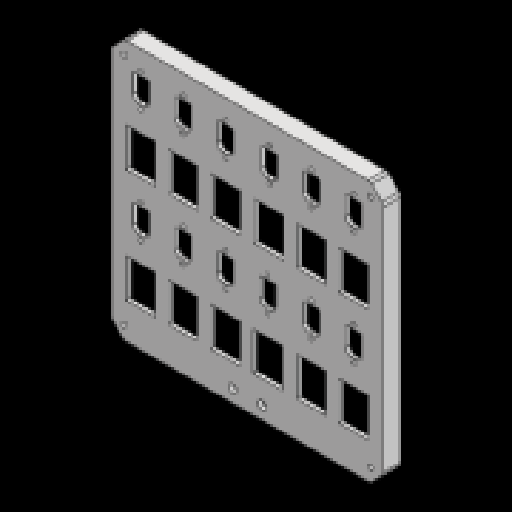
# Autodesk Inventor part: PowerHub
Saved by Autodesk Inventor 2025.2 (Build 292293000, 293)
## iProperties
Created: 2026-06-06
Part Number: PowerHub
Material: Generic
Document SubType Name: Modeling
Designer: valer
Density: 1 g/cm^3
Appearance: Default
Author: valer
Autodesk Inventor part; units mm, degrees
(part 1 of 2)
ref_plane "YZ Plane" through (0, 0, 0) normal (1, 0, 0) x (0, 1, 0)
ref_plane "XZ Plane" through (0, 0, 0) normal (0, 1, 0) x (-1, 0, 0)
ref_plane "XY Plane" through (0, 0, 0) normal (0, 0, 1) x (1, 0, 0)
sketch "Panel" plane through (0, 0, 0) normal (0, 0, 1) x (1, 0, 0)
  line L0 (-102.5, -98.125) -> (102.5, -98.125)
  line L1 (102.5, -98.125) -> (102.5, 98.125)
  line L2 (102.5, 98.125) -> (-102.5, 98.125)
  line L3 (-102.5, 98.125) -> (-102.5, -98.125)
  line L4 (-102.5, -98.125) -> (102.5, 98.125) construction
  line L5 (102.5, -98.125) -> (-102.5, 98.125) construction
  line L6 (-143.5, 0) -> (143.5, 0) construction
  line L7 (0, -137.375) -> (0, 137.375) construction
  line L8 (-88, 88.125) -> (-72, 88.125)
  line L9 (-72, 88.125) -> (-72, 54.125)
  line L10 (-72, 54.125) -> (-88, 54.125)
  line L11 (-88, 54.125) -> (-88, 88.125)
  line L12 (-80, 88.125) -> (-80, 12.875) construction
  line L13 (-92.5, 44.375) -> (-67.5, 44.375)
  line L14 (-67.5, 44.375) -> (-67.5, 12.875)
  line L15 (-67.5, 12.875) -> (-92.5, 12.875)
  line L16 (-92.5, 12.875) -> (-92.5, 44.375)
  line L17 (-56, 88.125) -> (-40, 88.125)
  line L18 (-56, 54.125) -> (-56, 88.125)
  line L19 (-40, 88.125) -> (-40, 54.125)
  line L20 (-40, 54.125) -> (-56, 54.125)
  line L21 (-60.5, 44.375) -> (-35.5, 44.375)
  line L22 (-60.5, 12.875) -> (-60.5, 44.375)
  line L23 (-35.5, 44.375) -> (-35.5, 12.875)
  line L24 (-35.5, 12.875) -> (-60.5, 12.875)
  line L25 (-24, 88.125) -> (-8, 88.125)
  line L26 (-24, 54.125) -> (-24, 88.125)
  line L27 (-8, 88.125) -> (-8, 54.125)
  line L28 (-8, 54.125) -> (-24, 54.125)
  line L29 (-28.5, 44.375) -> (-3.5, 44.375)
  line L30 (-28.5, 12.875) -> (-28.5, 44.375)
  line L31 (-3.5, 44.375) -> (-3.5, 12.875)
  line L32 (-3.5, 12.875) -> (-28.5, 12.875)
  line L33 (8, 88.125) -> (24, 88.125)
  line L34 (8, 54.125) -> (8, 88.125)
  line L35 (24, 88.125) -> (24, 54.125)
  line L36 (24, 54.125) -> (8, 54.125)
  line L37 (3.5, 44.375) -> (28.5, 44.375)
  line L38 (3.5, 12.875) -> (3.5, 44.375)
  line L39 (28.5, 44.375) -> (28.5, 12.875)
  line L40 (28.5, 12.875) -> (3.5, 12.875)
  line L41 (40, 88.125) -> (56, 88.125)
  line L42 (40, 54.125) -> (40, 88.125)
  line L43 (56, 88.125) -> (56, 54.125)
  line L44 (56, 54.125) -> (40, 54.125)
  line L45 (35.5, 44.375) -> (60.5, 44.375)
  line L46 (35.5, 12.875) -> (35.5, 44.375)
  line L47 (60.5, 44.375) -> (60.5, 12.875)
  line L48 (60.5, 12.875) -> (35.5, 12.875)
  line L49 (72, 88.125) -> (88, 88.125)
  line L50 (72, 54.125) -> (72, 88.125)
  line L51 (88, 88.125) -> (88, 54.125)
  line L52 (88, 54.125) -> (72, 54.125)
  line L53 (67.5, 44.375) -> (92.5, 44.375)
  line L54 (67.5, 12.875) -> (67.5, 44.375)
  line L55 (92.5, 44.375) -> (92.5, 12.875)
  line L56 (92.5, 12.875) -> (67.5, 12.875)
  line L57 (-88, 3.125) -> (-72, 3.125)
  line L58 (-88, -30.875) -> (-88, 3.125)
  line L59 (-72, 3.125) -> (-72, -30.875)
  line L60 (-72, -30.875) -> (-88, -30.875)
  line L61 (-92.5, -40.625) -> (-67.5, -40.625)
  line L62 (-92.5, -72.125) -> (-92.5, -40.625)
  line L63 (-67.5, -40.625) -> (-67.5, -72.125)
  line L64 (-67.5, -72.125) -> (-92.5, -72.125)
  line L65 (-56, 3.125) -> (-40, 3.125)
  line L66 (-56, -30.875) -> (-56, 3.125)
  line L67 (-40, 3.125) -> (-40, -30.875)
  line L68 (-40, -30.875) -> (-56, -30.875)
  line L69 (-60.5, -40.625) -> (-35.5, -40.625)
  line L70 (-60.5, -72.125) -> (-60.5, -40.625)
  line L71 (-35.5, -40.625) -> (-35.5, -72.125)
  line L72 (-35.5, -72.125) -> (-60.5, -72.125)
  line L73 (-24, 3.125) -> (-8, 3.125)
  line L74 (-24, -30.875) -> (-24, 3.125)
  line L75 (-8, 3.125) -> (-8, -30.875)
  line L76 (-8, -30.875) -> (-24, -30.875)
  line L77 (-28.5, -40.625) -> (-3.5, -40.625)
  line L78 (-28.5, -72.125) -> (-28.5, -40.625)
  line L79 (-3.5, -40.625) -> (-3.5, -72.125)
  line L80 (-3.5, -72.125) -> (-28.5, -72.125)
  line L81 (8, 3.125) -> (24, 3.125)
  line L82 (8, -30.875) -> (8, 3.125)
  line L83 (24, 3.125) -> (24, -30.875)
  line L84 (24, -30.875) -> (8, -30.875)
  line L85 (3.5, -40.625) -> (28.5, -40.625)
  line L86 (3.5, -72.125) -> (3.5, -40.625)
  line L87 (28.5, -40.625) -> (28.5, -72.125)
  line L88 (28.5, -72.125) -> (3.5, -72.125)
  line L89 (40, 3.125) -> (56, 3.125)
  line L90 (40, -30.875) -> (40, 3.125)
  line L91 (56, 3.125) -> (56, -30.875)
  line L92 (56, -30.875) -> (40, -30.875)
  line L93 (35.5, -40.625) -> (60.5, -40.625)
  line L94 (35.5, -72.125) -> (35.5, -40.625)
  line L95 (60.5, -40.625) -> (60.5, -72.125)
  line L96 (60.5, -72.125) -> (35.5, -72.125)
  line L97 (72, 3.125) -> (88, 3.125)
  line L98 (72, -30.875) -> (72, 3.125)
  line L99 (88, 3.125) -> (88, -30.875)
  line L100 (88, -30.875) -> (72, -30.875)
  line L101 (67.5, -40.625) -> (92.5, -40.625)
  line L102 (67.5, -72.125) -> (67.5, -40.625)
  line L103 (92.5, -40.625) -> (92.5, -72.125)
  line L104 (92.5, -72.125) -> (67.5, -72.125)
  line L105 (-11, -88.625) -> (11, -88.625) construction
  circle A0 centre (-11, -88.625) radius 3.2
  circle A1 centre (11, -88.625) radius 3.2
  line L106 (-20.5, -98.125) -> (-1.5, -98.125)
  line L107 (-1.5, -98.125) -> (-1.5, -79.125)
  line L108 (-1.5, -79.125) -> (-20.5, -79.125)
  line L109 (-20.5, -79.125) -> (-20.5, -98.125)
  line L110 (-20.5, -98.125) -> (-1.5, -79.125) construction
  line L111 (-1.5, -98.125) -> (-20.5, -79.125) construction
  line L112 (1.5, -98.125) -> (20.5, -98.125)
  line L113 (20.5, -98.125) -> (20.5, -79.125)
  line L114 (20.5, -79.125) -> (1.5, -79.125)
  line L115 (1.5, -79.125) -> (1.5, -98.125)
  line L116 (1.5, -98.125) -> (20.5, -79.125) construction
  line L117 (20.5, -98.125) -> (1.5, -79.125) construction
  line L118 (-22.5, -77.125) -> (22.5, -77.125)
  line L119 (22.5, -77.125) -> (22.5, -98.125)
  line L120 (22.5, -98.125) -> (-22.5, -98.125)
  line L121 (-22.5, -98.125) -> (-22.5, -77.125)
  point P0 (0, 0)
  point P1 (-48, 88.125)
  point P2 (-48, 12.875)
  point P3 (-16, 88.125)
  point P4 (-16, 12.875)
  point P5 (16, 88.125)
  point P6 (16, 12.875)
  point P7 (48, 88.125)
  point P8 (48, 12.875)
  point P9 (80, 88.125)
  point P10 (80, 12.875)
  point P11 (-80, 3.125)
  point P12 (-80, -72.125)
  point P13 (-48, 3.125)
  point P14 (-48, -72.125)
  point P15 (-16, 3.125)
  point P16 (-16, -72.125)
  point P17 (16, 3.125)
  point P18 (16, -72.125)
  point P19 (48, 3.125)
  point P20 (48, -72.125)
  point P21 (80, 3.125)
  point P22 (80, -72.125)
  point P23 (0, -88.625)
  dimension "d0" = 16
  dimension "d1" = 34
  dimension "d2" = 25
  dimension "d3" = 31.5
  dimension "d4" = 9.75
  dimension "d5" = 10
  dimension "d6" = 10
  dimension "d9" = 32
  dimension "d12" = 85
  dimension "d15" = 10
  dimension "d16" = 9.75
  dimension "d17" = 22
  dimension "d18" = 6.4
  dimension "d19" = 19
  dimension "d24" = 2
  dimension "d25" = 2
  dimension "d26" = 2
  dimension "d27" = 5
  dimension "d37" = 16
  dimension "d38" = 14.5
  constraints: 240 end point, 12 parallel, 9 midpoint, 8 horizontal, 7 perpendicular, 4 collinear, 3 equal length, 2 centre point, 2 coincident, 1 equal radius, 1 point on line, 1 vertical, 196 other
  measures "d0" distance of L8.start L8.end
  measures "d1" distance of L8.end L9.end
  measures "d2" distance of L14.end L15.end
  measures "d3" distance of L13.end L14.end
  measures "d4" distance between parallel lines of L13 L10
  measures "d5" distance between parallel lines of L3 L16
  measures "d6" distance between parallel lines of L2 L8
  measures "d9" distance of L8.start L17.start
  measures "d12" distance of L8.start L57.start
  measures "d15" distance between parallel lines of L1 L55
  measures "d16" distance between parallel lines of L57 L15
  measures "d17" distance of L105.start L105.end
  measures "d18" diameter of A0
  measures "d19" distance of L107.end L108.end
  measures "d24" distance between parallel lines of L118 L114
  measures "d25" distance between parallel lines of L119 L113
  measures "d26" distance between parallel lines of L109 L121
  measures "d27" distance between parallel lines of L118 L80
  measures "d37" distance between parallel lines of L18 L9
  measures "d38" distance between parallel lines of L3 L11
extrude "PanelFeature" add sketch "Panel" along normal blind 3 contours L3 L2 L1 L0 L119 L118 L121 | L121 L118 L119 L0 L113 L114 L115 L107 L108 L109 | L109 L108 L107 L0 | L115 L114 L113 L0 | L8 L9 L10 L11 | L13 L14 L15 L16 | L17 L19 L20 L18 | L21 L23 L24 L22 | L25 L27 L28 L26 | L29 L31 L32 L30 | L33 L35 L36 L34 | L37 L39 L40 L38 | L41 L43 L44 L42 | L45 L47 L48 L46 | L49 L51 L52 L50 | L53 L55 L56 L54 | L57 L59 L60 L58 | L61 L63 L64 L62 | L65 L67 L68 L66 | L69 L71 L72 L70 | L73 L75 L76 L74 | L77 L79 L80 L78 | L81 L83 L84 L82 | L85 L87 L88 L86 | L89 L91 L92 L90 | L93 L95 L96 L94 | L97 L99 L100 L98 | L101 L103 L104 L102
chamfer "OutsideChamfersFeature" distance 10 angle 45 4 edges at (-102.5, 98.125, 1.5) (-102.5, -98.125, 1.5) (102.5, -98.125, 1.5) (102.5, 98.125, 1.5)
fillet "FilletsFeature" radius 4 8 edges at (-92.5, -98.125, 1.5) (-102.5, -88.125, 1.5) (92.5, -98.125, 1.5) (102.5, -88.125, 1.5) (92.5, 98.125, 1.5) (102.5, 88.125, 1.5) (-102.5, 88.125, 1.5) (-92.5, 98.125, 1.5)
sketch "MountHoles" plane through (0, 0, 3) normal (0, 0, 1) x (1, 0, 0)
  arc A0 (-90.8431, 98.125) -> (-93.6716, 96.9534) centre (-90.8431, 94.125) ccw projected
  line L0 (-101.3284, 89.2966) -> (-93.6716, 96.9534) projected
  arc A1 (-101.3284, 89.2966) -> (-102.5, 86.4681) centre (-98.5, 86.4681) ccw projected
  line L1 (-102.5, 86.4681) -> (-102.5, -86.4681) projected
  arc A2 (-102.5, -86.4681) -> (-101.3284, -89.2966) centre (-98.5, -86.4681) ccw projected
  line L2 (-93.6716, -96.9534) -> (-101.3284, -89.2966) projected
  arc A3 (-93.6716, -96.9534) -> (-90.8431, -98.125) centre (-90.8431, -94.125) ccw projected
  line L3 (-90.8431, -98.125) -> (90.8431, -98.125) projected
  arc A4 (90.8431, -98.125) -> (93.6716, -96.9534) centre (90.8431, -94.125) ccw projected
  line L4 (101.3284, -89.2966) -> (93.6716, -96.9534) projected
  arc A5 (101.3284, -89.2966) -> (102.5, -86.4681) centre (98.5, -86.4681) ccw projected
  line L5 (102.5, -86.4681) -> (102.5, 86.4681) projected
  arc A6 (102.5, 86.4681) -> (101.3284, 89.2966) centre (98.5, 86.4681) ccw projected
  line L6 (93.6716, 96.9534) -> (101.3284, 89.2966) projected
  arc A7 (93.6716, 96.9534) -> (90.8431, 98.125) centre (90.8431, 94.125) ccw projected
  line L7 (90.8431, 98.125) -> (-90.8431, 98.125) projected
  circle A8 centre (-92.5, 88.125) radius 2
  line L8 (-143.8938, 0) -> (143.8938, 0) projected
  line L9 (0, -137.7688) -> (0, 137.7688) projected
  circle A9 centre (92.5, 88.125) radius 2
  circle A10 centre (-92.5, -88.125) radius 2
  circle A11 centre (92.5, -88.125) radius 2
  point P0 (0, 0)
  dimension "d32" = 4
  dimension "d33" = 10
  dimension "d34" = 10
  constraints: 4 centre point, 3 symmetric about line, 3 other
  measures "d32" diameter of A8
  measures "d33" distance from line of L7 A8.centre
  measures "d34" distance from line of L1 A8.centre
extrude "MountHolesFeature" cut sketch "MountHoles" against normal through all contours A8 | A9 | A10 | A11
sketch "ThroughHoles" plane through (0, 0, 0) normal (0, 0, -1) x (-1, 0, 0)
  circle A0 centre (-80.1, 67.625) radius 2.5 projected
  circle A1 centre (-80.1, 74.625) radius 2.5 projected
  arc A2 (-86, 65.675) -> (-82.2, 61.875) centre (-82.2, 65.675) ccw projected
  line L0 (-82.2, 61.875) -> (-78, 61.875) projected
  arc A3 (-78, 61.875) -> (-74.2, 65.675) centre (-78, 65.675) ccw projected
  line L1 (-74.2, 65.675) -> (-74.2, 79.375) projected
  arc A4 (-74.2, 79.375) -> (-75.2, 80.375) centre (-75.2, 79.375) ccw projected
  line L2 (-75.2, 80.375) -> (-85, 80.375) projected
  arc A5 (-85, 80.375) -> (-86, 79.375) centre (-85, 79.375) ccw projected
  line L3 (-86, 79.375) -> (-86, 65.675) projected
  circle A6 centre (-48.3, 67.625) radius 2.5 projected
  circle A7 centre (-48.3, 74.625) radius 2.5 projected
  arc A8 (-54.2, 65.675) -> (-50.4, 61.875) centre (-50.4, 65.675) ccw projected
  line L4 (-50.4, 61.875) -> (-46.2, 61.875) projected
  arc A9 (-46.2, 61.875) -> (-42.4, 65.675) centre (-46.2, 65.675) ccw projected
  line L5 (-42.4, 65.675) -> (-42.4, 79.375) projected
  arc A10 (-42.4, 79.375) -> (-43.4, 80.375) centre (-43.4, 79.375) ccw projected
  line L6 (-43.4, 80.375) -> (-53.2, 80.375) projected
  arc A11 (-53.2, 80.375) -> (-54.2, 79.375) centre (-53.2, 79.375) ccw projected
  line L7 (-54.2, 79.375) -> (-54.2, 65.675) projected
  circle A12 centre (-16.5, 67.625) radius 2.5 projected
  circle A13 centre (-16.5, 74.625) radius 2.5 projected
  arc A14 (-22.4, 65.675) -> (-18.6, 61.875) centre (-18.6, 65.675) ccw projected
  line L8 (-18.6, 61.875) -> (-14.4, 61.875) projected
  arc A15 (-14.4, 61.875) -> (-10.6, 65.675) centre (-14.4, 65.675) ccw projected
  line L9 (-10.6, 65.675) -> (-10.6, 79.375) projected
  arc A16 (-10.6, 79.375) -> (-11.6, 80.375) centre (-11.6, 79.375) ccw projected
  line L10 (-11.6, 80.375) -> (-21.4, 80.375) projected
  arc A17 (-21.4, 80.375) -> (-22.4, 79.375) centre (-21.4, 79.375) ccw projected
  line L11 (-22.4, 79.375) -> (-22.4, 65.675) projected
  circle A18 centre (16.5, 67.625) radius 2.5 projected
  circle A19 centre (16.5, 74.625) radius 2.5 projected
  arc A20 (10.6, 65.675) -> (14.4, 61.875) centre (14.4, 65.675) ccw projected
  line L12 (14.4, 61.875) -> (18.6, 61.875) projected
  arc A21 (18.6, 61.875) -> (22.4, 65.675) centre (18.6, 65.675) ccw projected
  line L13 (22.4, 65.675) -> (22.4, 79.375) projected
  arc A22 (22.4, 79.375) -> (21.4, 80.375) centre (21.4, 79.375) ccw projected
  line L14 (21.4, 80.375) -> (11.6, 80.375) projected
  arc A23 (11.6, 80.375) -> (10.6, 79.375) centre (11.6, 79.375) ccw projected
  line L15 (10.6, 79.375) -> (10.6, 65.675) projected
  circle A24 centre (48.3, 67.625) radius 2.5 projected
  circle A25 centre (48.3, 74.625) radius 2.5 projected
  arc A26 (42.4, 65.675) -> (46.2, 61.875) centre (46.2, 65.675) ccw projected
  line L16 (46.2, 61.875) -> (50.4, 61.875) projected
  arc A27 (50.4, 61.875) -> (54.2, 65.675) centre (50.4, 65.675) ccw projected
  line L17 (54.2, 65.675) -> (54.2, 79.375) projected
  arc A28 (54.2, 79.375) -> (53.2, 80.375) centre (53.2, 79.375) ccw projected
  line L18 (53.2, 80.375) -> (43.4, 80.375) projected
  arc A29 (43.4, 80.375) -> (42.4, 79.375) centre (43.4, 79.375) ccw projected
  line L19 (42.4, 79.375) -> (42.4, 65.675) projected
  circle A30 centre (80.1, 67.625) radius 2.5 projected
  circle A31 centre (80.1, 74.625) radius 2.5 projected
  arc A32 (74.2, 65.675) -> (78, 61.875) centre (78, 65.675) ccw projected
  line L20 (78, 61.875) -> (82.2, 61.875) projected
  arc A33 (82.2, 61.875) -> (86, 65.675) centre (82.2, 65.675) ccw projected
  line L21 (86, 65.675) -> (86, 79.375) projected
  arc A34 (86, 79.375) -> (85, 80.375) centre (85, 79.375) ccw projected
  line L22 (85, 80.375) -> (75.2, 80.375) projected
  arc A35 (75.2, 80.375) -> (74.2, 79.375) centre (75.2, 79.375) ccw projected
  line L23 (74.2, 79.375) -> (74.2, 65.675) projected
  line L24 (73.4544, 40.127) -> (86.7456, 40.127) projected
  line L25 (86.7456, 40.127) -> (86.7456, 17.127) projected
  line L26 (86.7456, 17.127) -> (73.4544, 17.127) projected
  line L27 (73.4544, 17.127) -> (73.4544, 40.127) projected
  line L28 (90.895, 42.851) -> (69.305, 42.851) projected
  line L29 (69.305, 42.851) -> (69.305, 14.403) projected
  line L30 (69.305, 14.403) -> (90.895, 14.403) projected
  line L31 (90.895, 14.403) -> (90.895, 42.851) projected
  line L32 (41.6544, 40.127) -> (54.9456, 40.127) projected
  line L33 (54.9456, 40.127) -> (54.9456, 17.127) projected
  line L34 (54.9456, 17.127) -> (41.6544, 17.127) projected
  line L35 (41.6544, 17.127) -> (41.6544, 40.127) projected
  line L36 (59.095, 42.851) -> (37.505, 42.851) projected
  line L37 (37.505, 42.851) -> (37.505, 14.403) projected
  line L38 (37.505, 14.403) -> (59.095, 14.403) projected
  line L39 (59.095, 14.403) -> (59.095, 42.851) projected
  line L40 (9.8544, 40.127) -> (23.1456, 40.127) projected
  line L41 (23.1456, 40.127) -> (23.1456, 17.127) projected
  line L42 (23.1456, 17.127) -> (9.8544, 17.127) projected
  line L43 (9.8544, 17.127) -> (9.8544, 40.127) projected
  line L44 (27.295, 42.851) -> (5.705, 42.851) projected
  line L45 (5.705, 42.851) -> (5.705, 14.403) projected
  line L46 (5.705, 14.403) -> (27.295, 14.403) projected
  line L47 (27.295, 14.403) -> (27.295, 42.851) projected
  line L48 (-23.1456, 40.127) -> (-9.8544, 40.127) projected
  line L49 (-9.8544, 40.127) -> (-9.8544, 17.127) projected
  line L50 (-9.8544, 17.127) -> (-23.1456, 17.127) projected
  line L51 (-23.1456, 17.127) -> (-23.1456, 40.127) projected
  line L52 (-5.705, 42.851) -> (-27.295, 42.851) projected
  line L53 (-27.295, 42.851) -> (-27.295, 14.403) projected
  line L54 (-27.295, 14.403) -> (-5.705, 14.403) projected
  line L55 (-5.705, 14.403) -> (-5.705, 42.851) projected
  line L56 (-54.9456, 40.127) -> (-41.6544, 40.127) projected
  line L57 (-41.6544, 40.127) -> (-41.6544, 17.127) projected
  line L58 (-41.6544, 17.127) -> (-54.9456, 17.127) projected
  line L59 (-54.9456, 17.127) -> (-54.9456, 40.127) projected
  line L60 (-37.505, 42.851) -> (-59.095, 42.851) projected
  line L61 (-59.095, 42.851) -> (-59.095, 14.403) projected
  line L62 (-59.095, 14.403) -> (-37.505, 14.403) projected
  line L63 (-37.505, 14.403) -> (-37.505, 42.851) projected
  line L64 (-86.7456, 40.127) -> (-73.4544, 40.127) projected
  line L65 (-73.4544, 40.127) -> (-73.4544, 17.127) projected
  line L66 (-73.4544, 17.127) -> (-86.7456, 17.127) projected
  line L67 (-86.7456, 17.127) -> (-86.7456, 40.127) projected
  line L68 (-69.305, 42.851) -> (-90.895, 42.851) projected
  line L69 (-90.895, 42.851) -> (-90.895, 14.403) projected
  line L70 (-90.895, 14.403) -> (-69.305, 14.403) projected
  line L71 (-69.305, 14.403) -> (-69.305, 42.851) projected
  circle A36 centre (-80.1, -17.621) radius 2.5 projected
  circle A37 centre (-80.1, -10.621) radius 2.5 projected
  arc A38 (-86, -19.571) -> (-82.2, -23.371) centre (-82.2, -19.571) ccw projected
  line L72 (-82.2, -23.371) -> (-78, -23.371) projected
  arc A39 (-78, -23.371) -> (-74.2, -19.571) centre (-78, -19.571) ccw projected
  line L73 (-74.2, -19.571) -> (-74.2, -5.871) projected
  arc A40 (-74.2, -5.871) -> (-75.2, -4.871) centre (-75.2, -5.871) ccw projected
  line L74 (-75.2, -4.871) -> (-85, -4.871) projected
  arc A41 (-85, -4.871) -> (-86, -5.871) centre (-85, -5.871) ccw projected
  line L75 (-86, -5.871) -> (-86, -19.571) projected
  circle A42 centre (-48.3, -17.621) radius 2.5 projected
  circle A43 centre (-48.3, -10.621) radius 2.5 projected
  arc A44 (-54.2, -19.571) -> (-50.4, -23.371) centre (-50.4, -19.571) ccw projected
  line L76 (-50.4, -23.371) -> (-46.2, -23.371) projected
  arc A45 (-46.2, -23.371) -> (-42.4, -19.571) centre (-46.2, -19.571) ccw projected
  line L77 (-42.4, -19.571) -> (-42.4, -5.871) projected
  arc A46 (-42.4, -5.871) -> (-43.4, -4.871) centre (-43.4, -5.871) ccw projected
  line L78 (-43.4, -4.871) -> (-53.2, -4.871) projected
  arc A47 (-53.2, -4.871) -> (-54.2, -5.871) centre (-53.2, -5.871) ccw projected
  line L79 (-54.2, -5.871) -> (-54.2, -19.571) projected
  circle A48 centre (-15.3, -17.621) radius 2.5 projected
  circle A49 centre (-15.3, -10.621) radius 2.5 projected
  arc A50 (-21.2, -19.571) -> (-17.4, -23.371) centre (-17.4, -19.571) ccw projected
  line L80 (-17.4, -23.371) -> (-13.2, -23.371) projected
  arc A51 (-13.2, -23.371) -> (-9.4, -19.571) centre (-13.2, -19.571) ccw projected
  line L81 (-9.4, -19.571) -> (-9.4, -5.871) projected
  arc A52 (-9.4, -5.871) -> (-10.4, -4.871) centre (-10.4, -5.871) ccw projected
  line L82 (-10.4, -4.871) -> (-20.2, -4.871) projected
  arc A53 (-20.2, -4.871) -> (-21.2, -5.871) centre (-20.2, -5.871) ccw projected
  line L83 (-21.2, -5.871) -> (-21.2, -19.571) projected
  circle A54 centre (16.5, -17.621) radius 2.5 projected
  circle A55 centre (16.5, -10.621) radius 2.5 projected
  arc A56 (10.6, -19.571) -> (14.4, -23.371) centre (14.4, -19.571) ccw projected
  line L84 (14.4, -23.371) -> (18.6, -23.371) projected
  arc A57 (18.6, -23.371) -> (22.4, -19.571) centre (18.6, -19.571) ccw projected
  line L85 (22.4, -19.571) -> (22.4, -5.871) projected
  arc A58 (22.4, -5.871) -> (21.4, -4.871) centre (21.4, -5.871) ccw projected
  line L86 (21.4, -4.871) -> (11.6, -4.871) projected
  arc A59 (11.6, -4.871) -> (10.6, -5.871) centre (11.6, -5.871) ccw projected
  line L87 (10.6, -5.871) -> (10.6, -19.571) projected
  circle A60 centre (48.3, -17.621) radius 2.5 projected
  circle A61 centre (48.3, -10.621) radius 2.5 projected
  arc A62 (42.4, -19.571) -> (46.2, -23.371) centre (46.2, -19.571) ccw projected
  line L88 (46.2, -23.371) -> (50.4, -23.371) projected
  arc A63 (50.4, -23.371) -> (54.2, -19.571) centre (50.4, -19.571) ccw projected
  line L89 (54.2, -19.571) -> (54.2, -5.871) projected
  arc A64 (54.2, -5.871) -> (53.2, -4.871) centre (53.2, -5.871) ccw projected
  line L90 (53.2, -4.871) -> (43.4, -4.871) projected
  arc A65 (43.4, -4.871) -> (42.4, -5.871) centre (43.4, -5.871) ccw projected
  line L91 (42.4, -5.871) -> (42.4, -19.571) projected
  circle A66 centre (80.1, -17.621) radius 2.5 projected
  circle A67 centre (80.1, -10.621) radius 2.5 projected
  arc A68 (74.2, -19.571) -> (78, -23.371) centre (78, -19.571) ccw projected
  line L92 (78, -23.371) -> (82.2, -23.371) projected
  arc A69 (82.2, -23.371) -> (86, -19.571) centre (82.2, -19.571) ccw projected
  line L93 (86, -19.571) -> (86, -5.871) projected
  arc A70 (86, -5.871) -> (85, -4.871) centre (85, -5.871) ccw projected
  line L94 (85, -4.871) -> (75.2, -4.871) projected
  arc A71 (75.2, -4.871) -> (74.2, -5.871) centre (75.2, -5.871) ccw projected
  line L95 (74.2, -5.871) -> (74.2, -19.571) projected
  line L96 (73.4544, -45.119) -> (86.7456, -45.119) projected
  line L97 (86.7456, -45.119) -> (86.7456, -68.119) projected
  line L98 (86.7456, -68.119) -> (73.4544, -68.119) projected
  line L99 (73.4544, -68.119) -> (73.4544, -45.119) projected
  line L100 (90.895, -42.395) -> (69.305, -42.395) projected
  line L101 (69.305, -42.395) -> (69.305, -70.843) projected
  line L102 (69.305, -70.843) -> (90.895, -70.843) projected
  line L103 (90.895, -70.843) -> (90.895, -42.395) projected
  line L104 (41.6544, -45.119) -> (54.9456, -45.119) projected
  line L105 (54.9456, -45.119) -> (54.9456, -68.119) projected
  line L106 (54.9456, -68.119) -> (41.6544, -68.119) projected
  line L107 (41.6544, -68.119) -> (41.6544, -45.119) projected
  line L108 (59.095, -42.395) -> (37.505, -42.395) projected
  line L109 (37.505, -42.395) -> (37.505, -70.843) projected
  line L110 (37.505, -70.843) -> (59.095, -70.843) projected
  line L111 (59.095, -70.843) -> (59.095, -42.395) projected
  line L112 (9.8544, -45.119) -> (23.1456, -45.119) projected
  line L113 (23.1456, -45.119) -> (23.1456, -68.119) projected
  line L114 (23.1456, -68.119) -> (9.8544, -68.119) projected
  line L115 (9.8544, -68.119) -> (9.8544, -45.119) projected
  line L116 (27.295, -42.395) -> (5.705, -42.395) projected
  line L117 (5.705, -42.395) -> (5.705, -70.843) projected
  line L118 (5.705, -70.843) -> (27.295, -70.843) projected
  line L119 (27.295, -70.843) -> (27.295, -42.395) projected
  line L120 (-21.9456, -45.119) -> (-8.6544, -45.119) projected
  line L121 (-8.6544, -45.119) -> (-8.6544, -68.119) projected
  line L122 (-8.6544, -68.119) -> (-21.9456, -68.119) projected
  line L123 (-21.9456, -68.119) -> (-21.9456, -45.119) projected
  line L124 (-4.505, -42.395) -> (-26.095, -42.395) projected
  line L125 (-26.095, -42.395) -> (-26.095, -70.843) projected
  line L126 (-26.095, -70.843) -> (-4.505, -70.843) projected
  line L127 (-4.505, -70.843) -> (-4.505, -42.395) projected
  line L128 (-54.9456, -45.119) -> (-41.6544, -45.119) projected
  line L129 (-41.6544, -45.119) -> (-41.6544, -68.119) projected
  line L130 (-41.6544, -68.119) -> (-54.9456, -68.119) projected
  line L131 (-54.9456, -68.119) -> (-54.9456, -45.119) projected
  line L132 (-37.505, -42.395) -> (-59.095, -42.395) projected
  line L133 (-59.095, -42.395) -> (-59.095, -70.843) projected
  line L134 (-59.095, -70.843) -> (-37.505, -70.843) projected
  line L135 (-37.505, -70.843) -> (-37.505, -42.395) projected
  line L136 (-86.7456, -45.119) -> (-73.4544, -45.119) projected
  line L137 (-73.4544, -45.119) -> (-73.4544, -68.119) projected
  line L138 (-73.4544, -68.119) -> (-86.7456, -68.119) projected
  line L139 (-86.7456, -68.119) -> (-86.7456, -45.119) projected
  line L140 (-69.305, -42.395) -> (-90.895, -42.395) projected
  line L141 (-90.895, -42.395) -> (-90.895, -70.843) projected
  line L142 (-90.895, -70.843) -> (-69.305, -70.843) projected
  line L143 (-69.305, -70.843) -> (-69.305, -42.395) projected
  line L144 (-73.95, 79.375) -> (-73.95, 65.675)
  arc A72 (-78, 61.625) -> (-73.95, 65.675) centre (-78, 65.675) ccw
  line L145 (-78, 61.625) -> (-82.2, 61.625)
  arc A73 (-86.25, 65.675) -> (-82.2, 61.625) centre (-82.2, 65.675) ccw
  line L146 (-86.25, 65.675) -> (-86.25, 79.375)
  arc A74 (-85, 80.625) -> (-86.25, 79.375) centre (-85, 79.375) ccw
  line L147 (-85, 80.625) -> (-75.2, 80.625)
  arc A75 (-73.95, 79.375) -> (-75.2, 80.625) centre (-75.2, 79.375) ccw
  line L148 (-53.2, 80.625) -> (-43.4, 80.625)
  arc A76 (-42.15, 79.375) -> (-43.4, 80.625) centre (-43.4, 79.375) ccw
  line L149 (-42.15, 79.375) -> (-42.15, 65.675)
  arc A77 (-46.2, 61.625) -> (-42.15, 65.675) centre (-46.2, 65.675) ccw
  line L150 (-46.2, 61.625) -> (-50.4, 61.625)
  arc A78 (-54.45, 65.675) -> (-50.4, 61.625) centre (-50.4, 65.675) ccw
  line L151 (-54.45, 65.675) -> (-54.45, 79.375)
  arc A79 (-53.2, 80.625) -> (-54.45, 79.375) centre (-53.2, 79.375) ccw
  line L152 (-21.4, 80.625) -> (-11.6, 80.625)
  arc A80 (-10.35, 79.375) -> (-11.6, 80.625) centre (-11.6, 79.375) ccw
  line L153 (-10.35, 79.375) -> (-10.35, 65.675)
  arc A81 (-14.4, 61.625) -> (-10.35, 65.675) centre (-14.4, 65.675) ccw
  line L154 (-14.4, 61.625) -> (-18.6, 61.625)
  arc A82 (-22.65, 65.675) -> (-18.6, 61.625) centre (-18.6, 65.675) ccw
  line L155 (-22.65, 65.675) -> (-22.65, 79.375)
  arc A83 (-21.4, 80.625) -> (-22.65, 79.375) centre (-21.4, 79.375) ccw
  line L156 (11.6, 80.625) -> (21.4, 80.625)
  arc A84 (22.65, 79.375) -> (21.4, 80.625) centre (21.4, 79.375) ccw
  line L157 (22.65, 79.375) -> (22.65, 65.675)
  arc A85 (18.6, 61.625) -> (22.65, 65.675) centre (18.6, 65.675) ccw
  line L158 (18.6, 61.625) -> (14.4, 61.625)
  arc A86 (10.35, 65.675) -> (14.4, 61.625) centre (14.4, 65.675) ccw
  line L159 (10.35, 65.675) -> (10.35, 79.375)
  arc A87 (11.6, 80.625) -> (10.35, 79.375) centre (11.6, 79.375) ccw
  line L160 (43.4, 80.625) -> (53.2, 80.625)
  arc A88 (54.45, 79.375) -> (53.2, 80.625) centre (53.2, 79.375) ccw
  line L161 (54.45, 79.375) -> (54.45, 65.675)
  arc A89 (50.4, 61.625) -> (54.45, 65.675) centre (50.4, 65.675) ccw
  line L162 (50.4, 61.625) -> (46.2, 61.625)
  arc A90 (42.15, 65.675) -> (46.2, 61.625) centre (46.2, 65.675) ccw
  line L163 (42.15, 65.675) -> (42.15, 79.375)
  arc A91 (43.4, 80.625) -> (42.15, 79.375) centre (43.4, 79.375) ccw
  line L164 (75.2, 80.625) -> (85, 80.625)
  arc A92 (86.25, 79.375) -> (85, 80.625) centre (85, 79.375) ccw
  line L165 (86.25, 79.375) -> (86.25, 65.675)
  arc A93 (82.2, 61.625) -> (86.25, 65.675) centre (82.2, 65.675) ccw
  line L166 (82.2, 61.625) -> (78, 61.625)
  arc A94 (73.95, 65.675) -> (78, 61.625) centre (78, 65.675) ccw
  line L167 (73.95, 65.675) -> (73.95, 79.375)
  arc A95 (75.2, 80.625) -> (73.95, 79.375) centre (75.2, 79.375) ccw
  line L168 (-69.055, 43.101) -> (-91.145, 43.101)
  line L169 (-91.145, 43.101) -> (-91.145, 14.153)
  line L170 (-91.145, 14.153) -> (-69.055, 14.153)
  line L171 (-69.055, 14.153) -> (-69.055, 43.101)
  line L172 (-59.345, 43.101) -> (-37.255, 43.101)
  line L173 (-37.255, 43.101) -> (-37.255, 14.153)
  line L174 (-37.255, 14.153) -> (-59.345, 14.153)
  line L175 (-59.345, 14.153) -> (-59.345, 43.101)
  line L176 (-27.545, 43.101) -> (-5.455, 43.101)
  line L177 (-5.455, 43.101) -> (-5.455, 14.153)
  line L178 (-5.455, 14.153) -> (-27.545, 14.153)
  line L179 (-27.545, 14.153) -> (-27.545, 43.101)
  line L180 (5.455, 43.101) -> (27.545, 43.101)
  line L181 (27.545, 43.101) -> (27.545, 14.153)
  line L182 (27.545, 14.153) -> (5.455, 14.153)
  line L183 (5.455, 14.153) -> (5.455, 43.101)
  line L184 (37.255, 43.101) -> (59.345, 43.101)
  line L185 (59.345, 43.101) -> (59.345, 14.153)
  line L186 (59.345, 14.153) -> (37.255, 14.153)
  line L187 (37.255, 14.153) -> (37.255, 43.101)
  line L188 (69.055, 43.101) -> (91.145, 43.101)
  line L189 (91.145, 43.101) -> (91.145, 14.153)
  line L190 (91.145, 14.153) -> (69.055, 14.153)
  line L191 (69.055, 14.153) -> (69.055, 43.101)
  line L192 (-73.95, -5.871) -> (-73.95, -19.571)
  arc A96 (-78, -23.621) -> (-73.95, -19.571) centre (-78, -19.571) ccw
  line L193 (-78, -23.621) -> (-82.2, -23.621)
  arc A97 (-86.25, -19.571) -> (-82.2, -23.621) centre (-82.2, -19.571) ccw
  line L194 (-86.25, -19.571) -> (-86.25, -5.871)
  arc A98 (-85, -4.621) -> (-86.25, -5.871) centre (-85, -5.871) ccw
  line L195 (-85, -4.621) -> (-75.2, -4.621)
  arc A99 (-73.95, -5.871) -> (-75.2, -4.621) centre (-75.2, -5.871) ccw
  line L196 (-53.2, -4.621) -> (-43.4, -4.621)
  arc A100 (-42.15, -5.871) -> (-43.4, -4.621) centre (-43.4, -5.871) ccw
  line L197 (-42.15, -5.871) -> (-42.15, -19.571)
  arc A101 (-46.2, -23.621) -> (-42.15, -19.571) centre (-46.2, -19.571) ccw
  line L198 (-46.2, -23.621) -> (-50.4, -23.621)
  arc A102 (-54.45, -19.571) -> (-50.4, -23.621) centre (-50.4, -19.571) ccw
  line L199 (-54.45, -19.571) -> (-54.45, -5.871)
  arc A103 (-53.2, -4.621) -> (-54.45, -5.871) centre (-53.2, -5.871) ccw
  line L200 (-20.2, -4.621) -> (-10.4, -4.621)
  arc A104 (-9.15, -5.871) -> (-10.4, -4.621) centre (-10.4, -5.871) ccw
  line L201 (-9.15, -5.871) -> (-9.15, -19.571)
  arc A105 (-13.2, -23.621) -> (-9.15, -19.571) centre (-13.2, -19.571) ccw
  line L202 (-13.2, -23.621) -> (-17.4, -23.621)
  arc A106 (-21.45, -19.571) -> (-17.4, -23.621) centre (-17.4, -19.571) ccw
  line L203 (-21.45, -19.571) -> (-21.45, -5.871)
  arc A107 (-20.2, -4.621) -> (-21.45, -5.871) centre (-20.2, -5.871) ccw
  line L204 (11.6, -4.621) -> (21.4, -4.621)
  arc A108 (22.65, -5.871) -> (21.4, -4.621) centre (21.4, -5.871) ccw
  line L205 (22.65, -5.871) -> (22.65, -19.571)
  arc A109 (18.6, -23.621) -> (22.65, -19.571) centre (18.6, -19.571) ccw
  line L206 (18.6, -23.621) -> (14.4, -23.621)
  arc A110 (10.35, -19.571) -> (14.4, -23.621) centre (14.4, -19.571) ccw
  line L207 (10.35, -19.571) -> (10.35, -5.871)
  arc A111 (11.6, -4.621) -> (10.35, -5.871) centre (11.6, -5.871) ccw
  line L208 (43.4, -4.621) -> (53.2, -4.621)
  arc A112 (54.45, -5.871) -> (53.2, -4.621) centre (53.2, -5.871) ccw
  line L209 (54.45, -5.871) -> (54.45, -19.571)
  arc A113 (50.4, -23.621) -> (54.45, -19.571) centre (50.4, -19.571) ccw
  line L210 (50.4, -23.621) -> (46.2, -23.621)
  arc A114 (42.15, -19.571) -> (46.2, -23.621) centre (46.2, -19.571) ccw
  line L211 (42.15, -19.571) -> (42.15, -5.871)
  arc A115 (43.4, -4.621) -> (42.15, -5.871) centre (43.4, -5.871) ccw
  line L212 (75.2, -4.621) -> (85, -4.621)
  arc A116 (86.25, -5.871) -> (85, -4.621) centre (85, -5.871) ccw
  line L213 (86.25, -5.871) -> (86.25, -19.571)
  arc A117 (82.2, -23.621) -> (86.25, -19.571) centre (82.2, -19.571) ccw
  line L214 (82.2, -23.621) -> (78, -23.621)
  arc A118 (73.95, -19.571) -> (78, -23.621) centre (78, -19.571) ccw
  line L215 (73.95, -19.571) -> (73.95, -5.871)
  arc A119 (75.2, -4.621) -> (73.95, -5.871) centre (75.2, -5.871) ccw
  line L216 (-91.145, -42.145) -> (-69.055, -42.145)
  line L217 (-69.055, -42.145) -> (-69.055, -71.093)
  line L218 (-69.055, -71.093) -> (-91.145, -71.093)
  line L219 (-91.145, -71.093) -> (-91.145, -42.145)
  line L220 (-59.345, -42.145) -> (-37.255, -42.145)
  line L221 (-37.255, -42.145) -> (-37.255, -71.093)
  line L222 (-37.255, -71.093) -> (-59.345, -71.093)
  line L223 (-59.345, -71.093) -> (-59.345, -42.145)
  line L224 (-26.345, -42.145) -> (-4.255, -42.145)
  line L225 (-4.255, -42.145) -> (-4.255, -71.093)
  line L226 (-4.255, -71.093) -> (-26.345, -71.093)
  line L227 (-26.345, -71.093) -> (-26.345, -42.145)
  line L228 (5.455, -42.145) -> (27.545, -42.145)
  line L229 (27.545, -42.145) -> (27.545, -71.093)
  line L230 (27.545, -71.093) -> (5.455, -71.093)
  line L231 (5.455, -71.093) -> (5.455, -42.145)
  line L232 (37.255, -42.145) -> (59.345, -42.145)
  line L233 (59.345, -42.145) -> (59.345, -71.093)
  line L234 (59.345, -71.093) -> (37.255, -71.093)
  line L235 (37.255, -71.093) -> (37.255, -42.145)
  line L236 (69.055, -42.145) -> (91.145, -42.145)
  line L237 (91.145, -42.145) -> (91.145, -71.093)
  line L238 (91.145, -71.093) -> (69.055, -71.093)
  line L239 (69.055, -71.093) -> (69.055, -42.145)
  point P0 (0, 0)
  dimension "d39" = 0.25
  dimension "d40" = 0.25
  dimension "d41" = 0.25
  dimension "d42" = 0.25
  dimension "d43" = 0.25
  dimension "d44" = 0.25
  dimension "d45" = 0.25
  dimension "d46" = 0.25
  dimension "d47" = 0.25
  dimension "d48" = 0.25
  dimension "d49" = 0.25
  dimension "d50" = 0.25
  dimension "d51" = 0.25
  dimension "d52" = 0.25
  dimension "d53" = 0.25
  dimension "d54" = 0.25
  dimension "d55" = 0.25
  dimension "d56" = 0.25
  dimension "d57" = 0.25
  dimension "d58" = 0.25
  dimension "d59" = 0.25
  dimension "d60" = 0.25
  dimension "d61" = 0.25
  dimension "d62" = 0.25
  constraints: 192 end point, 96 point on circle, 48 centre point, 120 other
  measures "d39" distance between parallel lines of L1 L144
  measures "d40" distance between parallel lines of L6 L148
  measures "d41" distance between parallel lines of L10 L152
  measures "d42" distance between parallel lines of L14 L156
  measures "d43" distance between parallel lines of L18 L160
  measures "d44" distance between parallel lines of L22 L164
  measures "d45" distance between parallel lines of L71 L171
  measures "d46" distance between parallel lines of L60 L172
  measures "d47" distance between parallel lines of L52 L176
  measures "d48" distance between parallel lines of L44 L180
  measures "d49" distance between parallel lines of L36 L184
  measures "d50" distance between parallel lines of L28 L188
  measures "d51" distance between parallel lines of L73 L192
  measures "d52" distance between parallel lines of L78 L196
  measures "d53" distance between parallel lines of L82 L200
  measures "d54" distance between parallel lines of L86 L204
  measures "d55" distance between parallel lines of L90 L208
  measures "d56" distance between parallel lines of L94 L212
  measures "d57" distance between parallel lines of L140 L216
  measures "d58" distance between parallel lines of L132 L220
  measures "d59" distance between parallel lines of L124 L224
  measures "d60" distance between parallel lines of L116 L228
  measures "d61" distance between parallel lines of L108 L232
  measures "d62" distance between parallel lines of L100 L236
extrude "ThroughHolesFeature" cut sketch "ThroughHoles" against normal through all contours A0 | A1 | L3 A5 L2 A4 L1 A3 L0 A2 | A6 | A7 | L7 A11 L6 A10 L5 A9 L4 A8 | A12 | A13 | L11 A17 L10 A16 L9 A15 L8 A14 | A18 | A19 | L15 A23 L14 A22 L13 A21 L12 A20 | A24 | A25 | L19 A29 L18 A28 L17 A27 L16 A26 | A30 | A31 | L23 A35 L22 A34 L21 A33 L20 A32 | L24 L25 L26 L27 | L31 L30 L29 L28 | L32 L33 L34 L35 | L39 L38 L37 L36 | L40 L41 L42 L43 | L47 L46 L45 L44 | L48 L49 L50 L51 | L55 L54 L53 L52 | L56 L57 L58 L59 | L63 L62 L61 L60 | L64 L65 L66 L67 | L71 L70 L69 L68 | A36 | A37 | L75 A41 L74 A40 L73 A39 L72 A38 | A42 | A43 | L79 A47 L78 A46 L77 A45 L76 A44 | A48 | A49 | L83 A53 L82 A52 L81 A51 L80 A50 | A54 | A55 | L87 A59 L86 A58 L85 A57 L84 A56 | A60 | A61 | L91 A65 L90 A64 L89 A63 L88 A62 | A66 | A67 | L95 A71 L94 A70 L93 A69 L92 A68 | L96 L97 L98 L99 | L103 L102 L101 L100 | L104 L105 L106 L107 | L111 L110 L109 L108 | L112 L113 L114 L115 | L119 L118 L117 L116 | L120 L121 L122 L123 | L127 L126 L125 L124 | L128 L129 L130 L131 | L135 L134 L133 L132 | L136 L137 L138 L139 | L143 L142 L141 L140 | L144 A72 L145 A73 L146 A74 L147 A75 | L148 A76 L149 A77 L150 A78 L151 A79 | L152 A80 L153 A81 L154 A82 L155 A83 | L156 A84 L157 A85 L158 A86 L159 A87 | L160 A88 L161 A89 L162 A90 L163 A91 | L164 A92 L165 A93 L166 A94 L167 A95 | L171 L170 L169 L168 | L172 L173 L174 L175 | L176 L177 L178 L179 | L180 L181 L182 L183 | L184 L185 L186 L187 | L188 L189 L190 L191 | L192 A96 L193 A97 L194 A98 L195 A99 | L196 A100 L197 A101 L198 A102 L199 A103 | L200 A104 L201 A105 L202 A106 L203 A107 | L204 A108 L205 A109 L206 A110 L207 A111 | L208 A112 L209 A113 L210 A114 L211 A115 | L212 A116 L213 A117 L214 A118 L215 A119 | L216 L217 L218 L219 | L220 L221 L222 L223 | L224 L225 L226 L227 | L228 L229 L230 L231 | L232 L233 L234 L235 | L236 L237 L238 L239
sketch "ConnectorMountHoles" plane through (0, 0, 3) normal (0, 0, 1) x (1, 0, 0)
  circle A0 centre (-80.1, 83.625) radius 1.55 projected
  circle A1 centre (-80.1, 58.625) radius 1.55 projected
  circle A2 centre (-48.3, 58.625) radius 1.55 projected
  circle A3 centre (-48.3, 83.625) radius 1.55 projected
  circle A4 centre (-16.5, 83.625) radius 1.55 projected
  circle A5 centre (-16.5, 58.625) radius 1.55 projected
  circle A6 centre (16.5, 83.625) radius 1.55 projected
  circle A7 centre (16.5, 58.625) radius 1.55 projected
  circle A8 centre (48.3, 83.625) radius 1.55 projected
  circle A9 centre (48.3, 58.625) radius 1.55 projected
  circle A10 centre (80.1, 83.625) radius 1.55 projected
  circle A11 centre (80.1, 58.625) radius 1.55 projected
  circle A12 centre (-80.1, -1.621) radius 1.55 projected
  circle A13 centre (-48.3, -1.621) radius 1.55 projected
  circle A14 centre (-16.5, -1.621) radius 1.55 projected
  circle A15 centre (15.3, -1.621) radius 1.55 projected
  circle A16 centre (48.3, -1.621) radius 1.55 projected
  circle A17 centre (80.1, -1.621) radius 1.55 projected
  circle A18 centre (80.1, -26.621) radius 1.55 projected
  circle A19 centre (48.3, -26.621) radius 1.55 projected
  circle A20 centre (15.3, -26.621) radius 1.55 projected
  circle A21 centre (-16.5, -26.621) radius 1.55 projected
  circle A22 centre (-48.3, -26.621) radius 1.55 projected
  circle A23 centre (-80.1, -26.621) radius 1.55 projected
  circle A24 centre (-80.1, 83.625) radius 1.25
  circle A25 centre (-48.3, 83.625) radius 1.25
  circle A26 centre (-16.5, 83.625) radius 1.25
  circle A27 centre (16.5, 83.625) radius 1.25
  circle A28 centre (48.3, 83.625) radius 1.25
  circle A29 centre (80.1, 83.625) radius 1.25
  circle A30 centre (80.1, 58.625) radius 1.25
  circle A31 centre (48.3, 58.625) radius 1.25
  circle A32 centre (16.5, 58.625) radius 1.25
  circle A33 centre (-16.5, 58.625) radius 1.25
  circle A34 centre (-80.1, -1.621) radius 1.25
  circle A35 centre (-80.1, 58.625) radius 1.25
  circle A36 centre (-48.3, 58.625) radius 1.25
  circle A37 centre (-48.3, -1.621) radius 1.25
  circle A38 centre (-16.5, -1.621) radius 1.25
  circle A39 centre (15.3, -1.621) radius 1.25
  circle A40 centre (48.3, -1.621) radius 1.25
  circle A41 centre (80.1, -1.621) radius 1.25
  circle A42 centre (80.1, -26.621) radius 1.25
  circle A43 centre (48.3, -26.621) radius 1.25
  circle A44 centre (15.3, -26.621) radius 1.25
  circle A45 centre (-16.5, -26.621) radius 1.25
  circle A46 centre (-48.3, -26.621) radius 1.25
  circle A47 centre (-80.1, -26.621) radius 1.25
  point P0 (0, 0)
  dimension "d65" = 2.5
  dimension "d66" = 0.3
  dimension "d67" = 0.3
  dimension "d68" = 0.3
  dimension "d69" = 0.3
  dimension "d70" = 0.3
  dimension "d71" = 0.3
  dimension "d72" = 0.3
  dimension "d73" = 0.3
  dimension "d74" = 0.3
  dimension "d75" = 0.3
  dimension "d76" = 0.3
  dimension "d77" = 0.3
  dimension "d78" = 0.3
  dimension "d79" = 0.3
  dimension "d80" = 0.3
  dimension "d81" = 0.3
  dimension "d82" = 0.3
  dimension "d83" = 0.3
  dimension "d84" = 0.3
  dimension "d85" = 0.3
  dimension "d86" = 0.3
  dimension "d87" = 0.3
  dimension "d88" = 0.3
  dimension "d89" = 0.3
  constraints: 24 centre point, 1 coincident
  measures "d65" diameter of A24
  measures "d66" radial gap between concentric circles of A0 A24
  measures "d67" radial gap between concentric circles of A3 A25
  measures "d68" radial gap between concentric circles of A4 A26
  measures "d69" radial gap between concentric circles of A6 A27
  measures "d70" radial gap between concentric circles of A8 A28
  measures "d71" radial gap between concentric circles of A10 A29
  measures "d72" radial gap between concentric circles of A11 A30
  measures "d73" radial gap between concentric circles of A9 A31
  measures "d74" radial gap between concentric circles of A7 A32
  measures "d75" radial gap between concentric circles of A5 A33
  measures "d76" radial gap between concentric circles of A12 A34
  measures "d77" radial gap between concentric circles of A1 A35
  measures "d78" radial gap between concentric circles of A2 A36
  measures "d79" radial gap between concentric circles of A13 A37
  measures "d80" radial gap between concentric circles of A14 A38
  measures "d81" radial gap between concentric circles of A15 A39
  measures "d82" radial gap between concentric circles of A16 A40
  measures "d83" radial gap between concentric circles of A17 A41
  measures "d84" radial gap between concentric circles of A18 A42
  measures "d85" radial gap between concentric circles of A19 A43
  measures "d86" radial gap between concentric circles of A20 A44
  measures "d87" radial gap between concentric circles of A21 A45
  measures "d88" radial gap between concentric circles of A22 A46
  measures "d89" radial gap between concentric circles of A23 A47
extrude "ConnectorMountHolesFeature" cut sketch "ConnectorMountHoles" against normal through all contours A0 | A1 | A2 | A3 | A4 | A5 | A6 | A7 | A8 | A9 | A10 | A11 | A12 | A13 | A14 | A15 | A16 | A17 | A18 | A19 | A20 | A21 | A22 | A23 | A24 | A25 | A26 | A27 | A28 | A29 | A30 | A31 | A32 | A33 | A34 | A35 | A36 | A37 | A38 | A39 | A40 | A41 | A42 | A43 | A44 | A45 | A46 | A47